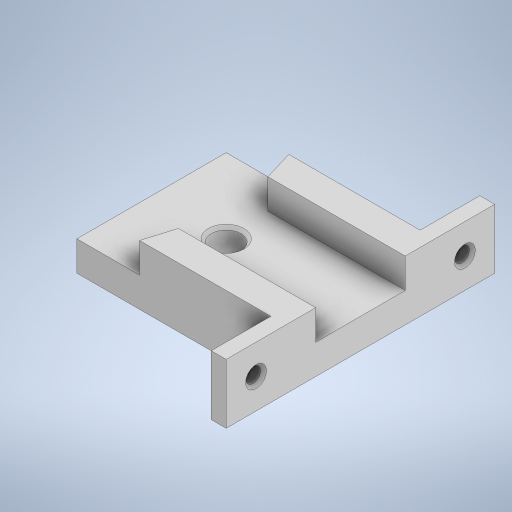
# Autodesk Inventor part: Стенка
Saved by Autodesk Inventor 2023 (Build 270158000, 158)
## iProperties
Created: 2022-04-28
Part Number: Стенка
Material: Типовые
Document SubType Name: Modeling
Designer: User
Density: 1 g/cm^3
Appearance: По умолчанию
Author: User
Autodesk Inventor part; units mm, degrees
ref_plane "YZ Plane" through (0, 0, 0) normal (1, 0, 0) x (0, 1, 0)
ref_plane "XZ Plane" through (0, 0, 0) normal (0, 1, 0) x (-1, 0, 0)
ref_plane "XY Plane" through (0, 0, 0) normal (0, 0, 1) x (1, 0, 0)
sketch "Эскиз1" plane through (0, 0, 0) normal (0, 1, 0) x (-1, 0, 0)
  line L0 (0, 0) -> (70, 0)
  line L1 (70, 0) -> (70, -50)
  line L2 (70, -50) -> (0, -50)
  line L3 (0, -50) -> (0, 0)
  dimension "d0" = 70
  dimension "d1" = 50
  constraints: 8 end point, 2 parallel, 1 horizontal, 1 perpendicular
  measures "d0" distance of L1.end L2.end
  measures "d1" distance of L0.end L1.end
extrude "Выдавливание1" add sketch "Эскиз1" along normal blind 10
sketch "Эскиз2" plane through (0, 10, 0) normal (0, 1, 0) x (1, 0, 0)
  line L0 (0, 0) -> (0, 50) projected
  line L1 (0, 25) -> (-45, 25)
  circle A0 centre (-45, 25) radius 5
  line L2 (0, 25) -> (0, 40)
  line L3 (0, 40) -> (-46, 40)
  line L4 (0, 25) -> (0, 10)
  line L5 (0, 10) -> (-46, 10)
  line L6 (-45, 25) -> (-70, 25)
  line L7 (-70, 50) -> (-70, 0) projected
  line L8 (-45, 25) -> (5, 25) construction
  line L9 (-45, 25) -> (-52.4371, 0.2096)
  line L10 (-45, 25) -> (15, 25) construction
  line L11 (-52.4371, 0.2096) -> (-52.4371, 49.7904)
  line L12 (-45, 25) -> (-52.4371, 49.7904)
  circle A1 centre (-45, 25) radius 9
  line L13 (-46, 40) -> (-49, 50)
  line L14 (-46, 10) -> (-49, 0)
  line L15 (-49, 0) -> (0, 0)
  line L16 (0, 0) -> (0, 50)
  line L17 (0, 50) -> (-49, 50)
  dimension "d4" = 45
  dimension "d5" = 10
  dimension "d6" = 15
  dimension "d7" = 15
  dimension "d12" = 146.602
  dimension "d13" = 18
  dimension "d18" = 49
  dimension "d19" = 46
  constraints: 32 end point, 4 perpendicular, 3 horizontal, 2 centre point, 2 coincident, 2 equal length, 2 midpoint, 2 parallel, 2 point on line, 1 vertical
  measures "d4" distance of L1.start L1.end
  measures "d5" diameter of A0
  measures "d6" distance of L1.start L2.end
  measures "d7" distance of L1.start L4.end
  measures "d12" angle of L9 L12
  measures "d13" diameter of A1
  measures "d18" distance of L0.end L13.end
  measures "d19" distance of L2.end L3.end
extrude "Выдавливание2" add sketch "Эскиз2" along normal blind 10 contours L15 L14 L5 L0 | L3 L13 L17 L0
extrude "Выдавливание3" cut sketch "Эскиз2" against normal blind 42.5 contours A0 L9 L1 | L1 L12 A0 | L9 A0 L6 | L6 A0 L12
sketch "Эскиз3" plane through (0, 0, 0) normal (0, -1, 0) x (1, 0, 0)
  circle A0 centre (-45, -25) radius 5 projected
  line L0 (-45, -25) -> (-15, -25)
  circle A1 centre (-15, -25) radius 6
  point P0 (0, 0)
  dimension "d20" = 30
  dimension "d21" = 12
  constraints: 2 end point, 1 centre point, 1 coincident, 1 horizontal
  measures "d20" distance of L0.start L0.end
  measures "d21" diameter of A1
extrude "Выдавливание4" cut sketch "Эскиз3" against normal blind 3 contours A1
chamfer "Фаска1" distance 1 angle 45 1 edges at (-21, 0, -25)
sketch "Эскиз4" plane through (0, 0, 0) normal (1, 0, 0) x (0, 0, -1)
  line L0 (0, 0) -> (0, 20) projected
  line L1 (0, 0) -> (-20, 0)
  line L2 (-20, 0) -> (-20, 20)
  line L3 (-20, 20) -> (0, 20)
  line L4 (0, 20) -> (0, 0)
  line L5 (50, 0) -> (50, 20) projected
  line L6 (50, 0) -> (70, 0)
  line L7 (70, 0) -> (70, 20)
  line L8 (70, 20) -> (50, 20)
  line L9 (50, 20) -> (50, 0)
  line L10 (70, 20) -> (60, 20)
  line L11 (60, 20) -> (60, 10)
  line L12 (60, 10) -> (70, 10)
  line L13 (70, 10) -> (70, 20)
  line L14 (-20, 20) -> (-10, 20)
  line L15 (-10, 20) -> (-10, 10)
  line L16 (-10, 10) -> (-20, 10)
  line L17 (-20, 10) -> (-20, 20)
  circle A0 centre (-10, 10) radius 2.5
  circle A1 centre (60, 10) radius 2.5
  line L18 (50, 20) -> (0, 20)
  dimension "d27" = 20
  dimension "d28" = 20
  dimension "d29" = 10
  dimension "d30" = 10
  dimension "d31" = 10
  dimension "d32" = 10
  dimension "d33" = 5
  dimension "d34" = 5
  constraints: 34 end point, 8 parallel, 5 perpendicular, 4 horizontal, 2 centre point, 2 coincident, 1 point on line
  measures "d27" distance of L2.end L3.end
  measures "d28" distance of L8.end L7.end
  measures "d29" distance of L12.end L11.end
  measures "d30" distance of L11.end L10.end
  measures "d31" distance of L15.end L16.end
  measures "d32" distance of L14.end L15.end
  measures "d33" diameter of A0
  measures "d34" diameter of A1
extrude "Выдавливание5" add sketch "Эскиз4" against normal blind 5 contours L1 L2 L16 A0 L15 L3 L0 | L15 A0 L16 L2 L3 | L5 L8 L11 A1 L12 L7 L6 | L8 L7 L12 A1 L11
chamfer "Фаска2" distance 1 angle 45 6 edges at (0, 10, -57.5) (0, 10, 12.5) (-5, 10, 12.5) (-5, 10, -57.5) (-50, 10, -25) (-50, 0, -25)
